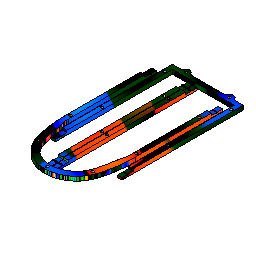
m365_bottom_ext2_5.5mm (Autodesk Fusion 360 design; units mm, degrees)
Autodesk Fusion 360 part; units mm, degrees
note: some values were not read from the file. Chosen so that the rebuilt part matches the saved one: which bodies a step acts on.
sketch "body" plane through (0, 0, 0) normal (0, 0, 1) x (1, 0, 0)
  arc A0 (-22.1801, -2.5) -> (-13.5199, -2.5) centre (-17.85, -5) cw
  arc A1 (-84.9273, -450.4931) -> (-79.697, -476.5511) centre (56.3, -435.6999) ccw
  circle A2 centre (-3, -100.5) radius 1.75
  circle A3 centre (-17.85, -5) radius 1.75
  arc A4 (-87.7, -435.6999) -> (-84.9273, -450.4931) centre (-46.85, -435.6999) ccw
  circle A5 centre (-82.35, -480.5) radius 1.75
  circle A6 centre (-90.7, -348) radius 1.75
  line L0 (-93.7, -435.6999) -> (-93.7, -5)
  line L1 (0, -5) -> (0, -435.6999)
  line L2 (-93.7, -5) -> (-84.5103, -5)
  line L3 (-87.7, -435.6999) -> (-87.7, -10.8)
  line L4 (-6, -435.6999) -> (-6, -10.8)
  line L5 (-9.1897, -5) -> (0, -5)
  line L6 (-67.1897, -5) -> (-26.5103, -5)
  line L7 (-6, -10.8) -> (-87.7, -10.8)
  circle A7 centre (-90.7, -265.5) radius 1.75
  circle A8 centre (-90.7, -430.5) radius 1.75
  arc A9 (-87.3378, -478.9225) -> (-93.7, -435.6999) centre (56.3, -435.6999) cw
  circle A10 centre (-11.35, -480.5) radius 1.75
  circle A11 centre (-3, -183.5) radius 1.75
  circle A12 centre (-90.7, -18) radius 1.75
  circle A13 centre (-90.7, -100.5) radius 1.75
  circle A14 centre (-90.7, -183.5) radius 1.75
  circle A15 centre (-3, -430.5) radius 1.75
  arc A16 (-13.5199, -2.5) -> (-9.1897, -5) centre (-9.1897, 0) ccw
  circle A17 centre (-3, -348) radius 1.75
  circle A18 centre (-75.85, -5) radius 1.75
  arc A19 (-8.7727, -450.4931) -> (-6, -435.6999) centre (-46.85, -435.6999) ccw
  arc A20 (-14.003, -476.5511) -> (-8.7727, -450.4931) centre (-150, -435.6999) ccw
  arc A21 (-84.5103, -5) -> (-80.1801, -2.5) centre (-84.5103, 0) ccw
  circle A22 centre (-3, -265.5) radius 1.75
  arc A23 (0, -435.6999) -> (-6.3622, -478.9225) centre (-150, -435.6999) cw
  arc A24 (-6.3622, -478.9225) -> (-87.3378, -478.9225) centre (-46.85, -466) cw
  circle A25 centre (-3, -18) radius 1.75
  arc A26 (-26.5103, -5) -> (-22.1801, -2.5) centre (-26.5103, 0) ccw
  circle A27 centre (-46.85, -504.5) radius 1.75
  arc A28 (-80.185, -474.8898) -> (-13.515, -474.8898) centre (-46.85, -466) ccw
  arc A29 (-71.5199, -2.5) -> (-67.1897, -5) centre (-67.1897, 0) ccw
  arc A30 (-80.1801, -2.5) -> (-71.5199, -2.5) centre (-75.85, -5) cw
  dimension "d1" = 5.8
  dimension "d2" = 6
  dimension "d3" = 6
  measures "d1" distance of L6 L7
  measures "d2" distance of L0 L3
  measures "d3" distance of L1 L4
extrude "Extrude1" add sketch "body" along normal blind 5.5 makes body 1
sketch "cuts" plane through (0, 0, 0) normal (1, 0, 0) x (0, 1, 0)
  line L0 (-5, 0) -> (-435.6999, 0)
  line L1 (-320, 0) -> (-320, 2.75)
  line L2 (-320, 2.75) -> (-327, 2.75)
  line L3 (-327, 2.75) -> (-327, 1.75)
  line L4 (-327, 1.75) -> (-328, 1.75)
  line L5 (-328, 1.75) -> (-328, 2.75)
  line L6 (-328, 2.75) -> (-335, 2.75)
  line L7 (-435.6999, 5.5) -> (-5, 5.5)
  line L8 (-335, 2.75) -> (-335, 5.5)
  line L9 (-165, 0) -> (-165, 2.75)
  line L10 (-165, 2.75) -> (-158, 2.75)
  line L11 (-158, 2.75) -> (-158, 1.75)
  line L12 (-158, 1.75) -> (-157, 1.75)
  line L13 (-157, 1.75) -> (-157, 2.75)
  line L14 (-157, 2.75) -> (-150, 2.75)
  line L15 (-150, 2.75) -> (-150, 5.5)
  dimension "d19" = 2.75
  dimension "d20" = 7
  dimension "d21" = 1
  dimension "d22" = 1
  dimension "d23" = 1
  dimension "d24" = 7
  dimension "d26" = 2.75
  dimension "d27" = 7
  dimension "d28" = 1
  dimension "d29" = 1
  dimension "d30" = 1
  dimension "d31" = 7
  measures "d26" distance of origin
split "Split1" by curves path "cuts" along L1 L2 L3 L4 L5 L6 L8 bodies 1 makes body 2 at (-3, -312.4167, 5.5)
split "Split2" by curves path "cuts" along L9 L10 L11 L12 L13 L14 L15 bodies 2 makes body 3 at (-3.061, -312.4135, 5.5) makes body 4 at (-2.9684, -144.0825, 0)
move_body "Move5" bodies 2 to x (-1, 0, 0) y (0, 1, 0) z (0, 0, -1) at (-175.4, 0, 5.5)
move_body "Move6" bodies 3 to x (-1, 0, 0) y (0, 1, 0) z (0, 0, -1) at (-12, 0, 5.5)
move_body "Move7" bodies 2 to x (1, 0, 0) y (0, 1, 0) z (0, 0, 1) at (34, -163, 0)
move_body "Move8" bodies 3 to x (1, 0, 0) y (0, 1, 0) z (0, 0, 1) at (-35, -163, 0)
move_body "Move9" bodies 4 to x (1, 0, 0) y (0, 1, 0) z (0, 0, 1) at (12, -300, 0)
equation "height = 5.5 mm"
equation "d5 = height"
equation "d19 = height / 2"
equation "d26 = height / 2"
